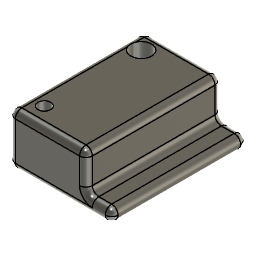
mpu mount (Autodesk Fusion 360 design; units mm, degrees)
part number: 2026-04-16-21-36-12-459
Autodesk Fusion 360 part; units mm, degrees
sketch "Main Body" plane through (0, 0, 0) normal (0, 0, 1) x (1, 0, 0)
  line L0 (0, 0) -> (16, 0)
  line L1 (16, 0) -> (16, 21.1)
  line L2 (16, 21.1) -> (0, 21.1)
  line L3 (0, 21.1) -> (0, 0)
  circle A0 centre (2.5, 18.1) radius 1.625
  line L4 (0, 10.55) -> (16, 10.55) construction
  circle A1 centre (2.5, 3) radius 1
  dimension "d1" = 16
  dimension "d2" = 21.1
  dimension "d3" = 3.25
  dimension "d4" = 3
  dimension "d5" = 2.5
  dimension "d6" = 10.55
  dimension "d11" = 2
  dimension "d12" = 2.5
  dimension "d13" = 3
  constraint horizontal L0
  constraint vertical L1
  constraint horizontal L2
  constraint vertical L3
  constraint coincident L0.start L3.end
  constraint coincident L3 L4.start
  constraint coincident L1 L4.end
  constraint perpendicular L1 L4
  measures "d1" distance of L1 L3
  measures "d2" distance of L0 L2
  measures "d3" diameter of A0
  measures "d4" distance of L2 A0.centre
  measures "d5" distance of L3 A0.centre
  measures "d6" distance of L0 L4
  measures "d11" diameter of A1
  measures "d12" distance of L3 A1.centre
  measures "d13" distance of L0 A1.centre
extrude "Extrude1" add sketch "Main Body" along normal blind 8
sketch "step_cut" plane through (0, 0, 8) normal (0, 0, 1) x (-1, 0, 0)
  circle A0 centre (-2.5, -3) radius 1
  circle A1 centre (-2.5, -18.1) radius 1.625
  line L0 (0, -21.1) -> (0, 0)
  line L1 (0, 0) -> (-16, 0)
  line L2 (-16, 0) -> (-16, -21.1)
  line L3 (-16, -21.1) -> (0, -21.1)
  line L4 (-16, -21.1) -> (-12, -21.1)
  line L5 (-12, -21.1) -> (-12, 0)
  line L6 (-12, 0) -> (-16, 0)
  line L7 (-16, 0) -> (-16, -21.1)
  constraint horizontal L4
  constraint vertical L5
  constraint horizontal L6
  constraint vertical L7
  constraint coincident L1 L5.end
  constraint coincident L2.end L3.start
extrude "Extrude2" cut sketch "step_cut" against normal blind 6 contours L1 L2 L3 L4 L5 L6 L7
fillet "Fillet1" radius 1 13 edges at (12, 10.55, 2) (12, 0, 5) (12, 21.1, 5) (0, 0, 4) (8, 0, 0) (16, 0, 1) (16, 21.1, 1) (16, 10.55, 0) (16, 10.55, 2) (14, 0, 2) (14, 21.1, 2) (12, 10.55, 8) (6, 0, 8) 2 faces at (0, 14.0667, 2.6667) (4, 21.1, 3.3333)
named bodies: "mpu_base_mount"
